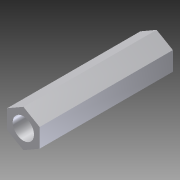
# Autodesk Inventor part: Stand offs BD motor mount
Saved by Autodesk Inventor 2012 (Build 160160000, 160)
## iProperties
Created: 2012-06-30
Part Number: Stand offs BD motor mount
Material: Default
Document SubType Name: Modeling
Designer: Bruce
Density: 1 g/cm^3
Author: Bruce
Autodesk Inventor part; units mm, degrees
ref_plane "YZ Plane" through (0, 0, 0) normal (1, 0, 0) x (0, 1, 0)
ref_plane "XZ Plane" through (0, 0, 0) normal (0, 1, 0) x (-1, 0, 0)
ref_plane "XY Plane" through (0, 0, 0) normal (0, 0, 1) x (1, 0, 0)
sketch "Sketch1" plane through (0, 0, 0) normal (0, 0, 1) x (1, 0, 0)
  circle A0 centre (0, 0) radius 3.81
  circle A1 centre (0, 0) radius 2.54
  line L0 (0, 4.4715) -> (3.8725, 2.2358)
  line L1 (3.8725, 2.2358) -> (3.8725, -2.2358)
  line L2 (3.8725, -2.2358) -> (0, -4.4715)
  line L3 (0, -4.4715) -> (-3.8725, -2.2358)
  line L4 (-3.8725, -2.2358) -> (-3.8725, 2.2358)
  line L5 (-3.8725, 2.2358) -> (0, 4.4715)
  dimension "d0" = 5.08
  dimension "d1" = 7.62
  constraints: 12 end point, 3 coincident, 2 centre point, 13 other
  measures "d0" diameter of A1
  measures "d1" diameter of A0
extrude "Extrusion1" add sketch "Sketch1" against normal blind 31.75 contours A0 | L0 L1 L2 L3 L4 L5
body "Solid1"
